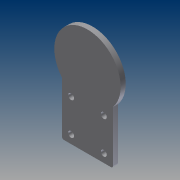
# Autodesk Inventor part: MotorMountTop
Saved by Autodesk Inventor 2011 SP1 (Build 150282100, 282)
## iProperties
Created: 2011-07-18
Part Number: MotorMountTop
Document SubType Name: Modeling
Designer: Nathan
Density: 1 g/cm^3
Author: Nathan
Autodesk Inventor part; units mm, degrees
ref_plane "YZ Plane" through (0, 0, 0) normal (1, 0, 0) x (0, 1, 0)
ref_plane "XZ Plane" through (0, 0, 0) normal (0, 1, 0) x (-1, 0, 0)
ref_plane "XY Plane" through (0, 0, 0) normal (0, 0, 1) x (1, 0, 0)
sketch "Sketch1" plane through (0, 0, 0) normal (0, 0, 1) x (1, 0, 0)
  line L0 (0, 0) -> (-14.605, 0)
  line L1 (-15.875, 1.27) -> (-15.875, 33.02)
  arc A0 (-15.875, 1.27) -> (-14.605, 0) centre (-14.605, 1.27) ccw
  line L2 (0, 11.7273) -> (0, 6.5424)
  line L3 (0, 0) -> (14.605, 0)
  line L4 (15.875, 1.27) -> (15.875, 33.02)
  arc A1 (14.605, 0) -> (15.875, 1.27) centre (14.605, 1.27) ccw
  arc A2 (15.875, 33.02) -> (-15.4781, 59.8572) centre (0, 46.2068) ccw
  arc A3 (-15.4781, 59.8572) -> (-15.875, 33.02) centre (0, 46.2068) ccw
  circle A4 centre (-10.16, 25.567) radius 1.8288
  circle A5 centre (10.16, 25.567) radius 1.8288
  circle A6 centre (-10.16, 5.247) radius 1.8288
  circle A7 centre (10.16, 5.247) radius 1.8288
  circle A8 centre (0, 46.2068) radius 6.35
  dimension "d1" = 14.605
  dimension "d2" = 1.27
  dimension "d4" = 31.75
  dimension "d8" = 31.75
  dimension "d42" = 20.6375
  dimension "d72" = 20.32
  dimension "d73" = 20.32
  dimension "d74" = 3.6576
  dimension "d75" = 3.6576
  dimension "d76" = 3.6576
  dimension "d77" = 3.6576
  dimension "d78" = 12.7
  constraints: 10 end point, 9 centre point, 8 point on circle, 5 coincident, 4 symmetric about line, 1 horizontal, 1 parallel, 1 perpendicular, 1 point on line, 1 other
  measures "d1" distance of L0.start L0.end
  measures "d2" horizontal distance of L0.end L1.start
  measures "d4" distance of L1.start L1.end
  measures "d8" distance between parallel lines of L1 L4
  measures "d42" radius of A3
  measures "d72" distance of point (10.16, 25.567) point (-10.16, 25.567)
  measures "d73" distance of point (10.16, 25.567) point (10.16, 5.247)
  measures "d74" diameter of A4
  measures "d75" diameter of A5
  measures "d76" diameter of A6
  measures "d77" diameter of A7
  measures "d78" diameter of A8
extrude "Extrusion1" add sketch "Sketch1" along normal blind 3.175 contours L0 A0 L1 A3 A2 L4 A1 L3 | A4 | A5 | A6 | A7 | A8
sketch "Sketch2" plane through (0, 0, 0) normal (0, 0, -1) x (-1, 0, 0)
  line L0 (-14.605, 0) -> (14.605, 0) projected
  arc A0 (15.875, 33.02) -> (-15.875, 33.02) centre (0, 46.2068) ccw projected
  line L1 (0, 46.2068) -> (15.24, 46.2068)
  line L2 (0, 46.2068) -> (0, 30.9668)
  line L3 (0, 46.2068) -> (0, 61.4468)
  line L4 (0, 46.2068) -> (-15.24, 46.2068)
  circle A1 centre (-10.16, 25.567) radius 1.8288
  circle A2 centre (10.16, 25.567) radius 1.8288
  circle A3 centre (-10.16, 5.247) radius 1.8288
  circle A4 centre (10.16, 5.247) radius 1.8288
  point P0 (0, 0)
  point P1 (15.875, 1.27)
  dimension "d52" = 15.24
  dimension "d53" = 15.24
  dimension "d54" = 15.24
  dimension "d55" = 15.24
  dimension "d58" = 31.75
  dimension "d59" = 13.1868
  dimension "d60" = 20.6375
  dimension "d61" = 46.2068
  dimension "d62" = 20.32
  dimension "d64" = 20.32
  dimension "d65" = 3.6576
  dimension "d67" = 3.6576
  dimension "d68" = 3.6576
  dimension "d69" = 3.6576
  constraints: 8 end point, 4 centre point, 4 coincident, 2 perpendicular, 2 symmetric about line, 1 collinear, 1 vertical
  measures "d52" distance of L1.start L4.end
  measures "d53" distance of L1.start L3.end
  measures "d54" distance of L1.start L1.end
  measures "d55" distance of L1.start L2.end
  measures "d58" distance of point (15.875, 1.27) A0.start
  measures "d59" vertical distance of A0.start L1.start
  measures "d60" radius of A0
  measures "d61" distance from line of L0 L1.start
  measures "d62" distance of point (10.16, 25.567) point (-10.16, 25.567)
  measures "d64" distance of point (10.16, 25.567) point (10.16, 5.247)
  measures "d65" diameter of A1
  measures "d67" diameter of A2
  measures "d68" diameter of A3
  measures "d69" diameter of A4
extrude "Extrusion2" cut sketch "Sketch2" against normal through all
body "Solid1"
